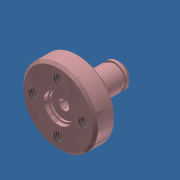
# Autodesk Inventor part: None_Magnet_Extender_Split_Top
Saved by Autodesk Inventor 2015 (Build 190159000, 159)
## iProperties
Created: 2015-01-06
Part Number: None_Magnet_Extender_Split_Top
Material: Aluminum 6061
Document SubType Name: Modeling
Designer: ice
Mass: 1.63117 g
Surface Area: 7.28726 cm^2
Volume: 0.604135 cm^3
Density: 2.7 g/cm^3
Appearance: Aluminum - Flat
Author: ice
Autodesk Inventor part; units mm, degrees
ref_plane "YZ Plane" through (0, 0, 0) normal (1, 0, 0) x (0, 1, 0)
sketch "Sketch1" plane through (0, 0, 0) normal (1, 0, 0) x (0, 1, 0)
  line L0 (31, 0) -> (20.4, 0)
  line L1 (31, 0) -> (32, 0)
  line L2 (32, 0) -> (32, 2.45)
  line L3 (32, 2.45) -> (30.5, 2.45)
  line L4 (30.5, 2.45) -> (30.5, 2.125)
  line L5 (30.5, 2.125) -> (29.7, 2.125)
  line L6 (29.7, 2.125) -> (29.7, 2.45)
  line L7 (29.7, 2.45) -> (26.7, 2.45)
  line L8 (26.7, 2.45) -> (26.7, 2.125)
  line L9 (26.7, 2.125) -> (25.9, 2.125)
  line L10 (25.9, 2.125) -> (25.9, 2.45)
  line L11 (25.9, 2.45) -> (24.4, 2.45)
  line L12 (23.4, 2.5) -> (24.4, 2.5)
  line L13 (24.4, 2.5) -> (24.4, 2.45)
  line L14 (23.4, 2.5) -> (23.4, 7.5)
  line L15 (32, 2.45) -> (31, 2.45)
  line L16 (32, 2.45) -> (32, 1.45)
  line L17 (19.6, 7.5) -> (23.4, 7.5)
  line L18 (20.4, 2.55) -> (20, 2.55)
  line L19 (19.2, 7.5) -> (19.6, 7.5)
  line L20 (20.4, 2.55) -> (20.4, 0)
  line L21 (20, 2.55) -> (20, 2.875)
  line L22 (20, 2.875) -> (19.2, 2.875)
  line L23 (19.2, 2.875) -> (19.2, 7.5)
  point P0 (0, 0)
  dimension "d344" = 1
  dimension "d345" = 1.5
  dimension "d346" = 0.325
  dimension "d347" = 0.8
  dimension "d348" = 3
  dimension "d349" = 0.325
  dimension "d350" = 0.8
  dimension "d351" = 2.45
  dimension "d353" = 1
  dimension "d354" = 1
  dimension "d355" = 1
  dimension "d377" = 0.4
  dimension "d379" = 2.55
  dimension "d380" = 0.8
  constraints: 48 end point, 8 perpendicular, 6 horizontal, 4 vertical, 3 point on line
  measures "d344" distance of L0.start L1.end
  measures "d345" distance of L2.end L3.end
  measures "d346" distance of L3.end L4.end
  measures "d347" distance of L4.end L5.end
  measures "d348" distance of L6.end L7.end
  measures "d349" distance of L7.end L8.end
  measures "d350" distance of L8.end L9.end
  measures "d351" distance between parallel lines of L0 L11
  measures "d353" distance of L12.start L12.end
  measures "d354" distance of L2.end L15.end
  measures "d355" distance of L2.end L16.end
  measures "d377" distance of L18.start L18.end
  measures "d379" distance of L0.end L18.start
  measures "d380" distance of L21.end L22.end
revolve "Revolution1" add sketch "Sketch1" angle 360 about axis through (0, 31, 0) along (0, -1, 0)
chamfer "Chamfer6" distance 0.5 angle 45 2 edges at (0, 23.4, -7.5) (0, 19.2, -7.5)
chamfer "Chamfer8" distance 1 angle 45 1 edges at (0, 32, -2.45)
sketch "Sketch13" plane through (0, 32, 0) normal (0, 1, 0) x (1, 0, 0)
  circle A0 centre (0, 0) radius 1
  point P0 (0, 0)
  dimension "d359" = 2
  constraints: 1 centre point, 1 coincident
  measures "d359" diameter of A0
hole "Hole10" at (0, 32, 0) direction (0, -1, 0) diameter 2 end through all
ref_plane "Work Plane8" through (0, 26.3, 0) normal (0, 1, 0) x (1, 0, 0)
ref_plane "Work Plane9" through (0, 30.1, 0) normal (0, 1, 0) x (1, 0, 0)
sketch "Sketch15" plane through (0, 19.2, 0) normal (0, -1, 0) x (1, 0, 0)
  line L0 (0, 0) -> (5, 0)
  line L1 (0, 0) -> (-5, 0)
  line L2 (0, 0) -> (0, -5)
  line L3 (0, 0) -> (0, 5)
  dimension "d381" = 5
  dimension "d382" = 5
  dimension "d383" = 5
  dimension "d384" = 5
  constraints: 8 end point, 2 horizontal, 2 vertical
  measures "d381" distance of L0.start L0.end
  measures "d382" distance of L0.start L1.end
  measures "d383" distance of L0.start L2.end
  measures "d384" distance of L0.start L3.end
hole "Hole11" at (0, 19.2, -5) at (-5, 19.2, 0) at (5, 19.2, 0) at (0, 19.2, 5) direction (0, 1, 0) diameter 1.9 end through all
thread "Thread21" size "M2x0.4" class "6H" standard "ANSI Metric M Profile" full length
thread "Thread22" size "M2x0.4" class "6H" standard "ANSI Metric M Profile" full length
thread "Thread23" size "M2x0.4" class "6H" standard "ANSI Metric M Profile" full length
thread "Thread24" size "M2x0.4" class "6H" standard "ANSI Metric M Profile" full length
body "Solid1"
